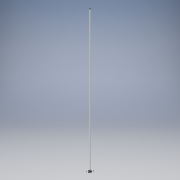
# Autodesk Inventor part: Tengely
Saved by Autodesk Inventor 2019 (Build 230136000, 136)
## iProperties
Created: 2020-01-23
Part Number: Tengely
Material: Generic
Document SubType Name: Modeling
Designer: laca
Density: 1 g/cm^3
Appearance: Default
Author: laca
Autodesk Inventor part; units mm, degrees
ref_plane "YZ Plane" through (0, 0, 0) normal (1, 0, 0) x (0, 1, 0)
ref_plane "XZ Plane" through (0, 0, 0) normal (0, 1, 0) x (-1, 0, 0)
ref_plane "XY Plane" through (0, 0, 0) normal (0, 0, 1) x (1, 0, 0)
sketch "Sketch1" plane through (0, 0, 0) normal (0, 1, 0) x (-1, 0, 0)
  circle A0 centre (0, 0) radius 7
  circle A1 centre (0, 0) radius 3
  dimension "d0" = 14
  dimension "d1" = 6
  constraints: 2 centre point, 2 coincident
  measures "d0" diameter of A0
  measures "d1" diameter of A1
extrude "Extrusion1" add sketch "Sketch1" along normal blind 1000 contours A0 | A1
extrude "Extrusion2" cut sketch "Sketch1" along normal blind 50 contours A1
chamfer "Chamfer1" distance 1 angle 45 1 edges at (7, 0, 0)
mirror "Mirror1" about plane through (0, 1000, 0) normal (0, 1, 0) of "Extrusion1", "Extrusion2", "Chamfer1"
body "Solid1"
